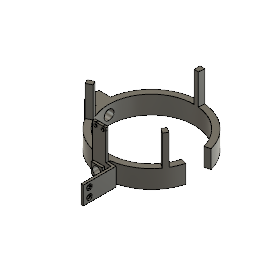
250-ml-band (Autodesk Fusion 360 design; units mm, degrees)
Autodesk Fusion 360 part; units mm, degrees
note: some values were not read from the file. Set by a fixed rule: which sketch regions a step uses.
sketch "Sketch1" plane through (0, 0, 0) normal (0, 1, 0) x (1, 0, 0)
  circle A0 centre (0, 0) radius 35
  circle A1 centre (0, 0) radius 40
  dimension "d1" = 70
  dimension "d2" = 5
  measures "d1" diameter of A0
extrude "Extrude1" add sketch "Sketch1" along normal blind 15
sketch "Sketch4" plane through (0, 15, 0) normal (0, 1, 0) x (-1, 0, 0)
  circle A0 centre (0, 0) radius 35
  circle A1 centre (0, 0) radius 40
  line L0 (0, 0) -> (0, -40)
  line L1 (0, 0) -> (-4.1811, -39.7809)
  line L2 (0, 0) -> (40, 0) construction
  dimension "d5" = 96
  dimension "d6" = 40
  measures "d5" angle of L1 L2
  measures "d6" distance of A0.centre L1.end
extrude "Extrude2" add sketch "Sketch4" along normal blind 25 contours A0 A1 L0 L1 picked at (-1.8026, -38.2856)
sketch "Sketch5" plane through (0, 15, 0) normal (0, 1, 0) x (-1, 0, 0)
  line L0 (0, -35) -> (0, -40)
  arc A0 (0, -40) -> (-4.1811, -39.7809) centre (0, 0) ccw
  line L1 (-4.1811, -39.7809) -> (-3.6585, -34.8083)
  arc A1 (0, -35) -> (-3.6585, -34.8083) centre (0, 0) ccw
  line L2 (0, 0) -> (-38.637, 10.3528)
  line L3 (0, 0) -> (40, 0) construction
  line L4 (0, 0) -> (-38.637, -10.3528)
  line L5 (0, 0) -> (-40, 0) construction
  dimension "d9" = 165
  dimension "d10" = 40
  dimension "d11" = 15
  dimension "d12" = 40
  measures "d9" angle of L2 L3
  measures "d10" distance of A0.centre L2.end
  measures "d11" angle of L4 L5
  measures "d12" distance of A0.centre L4.end
extrude "Extrude3" cut sketch "Sketch5" against normal blind 15 contours A0 A1 L2 L4
sketch "Sketch6" plane through (0, 15, 0) normal (0, 1, 0) x (-1, 0, 0)
  line L0 (-38.637, 10.3528) -> (-33.8074, 9.0587)
  arc A0 (0, -35) -> (-33.8074, 9.0587) centre (0, 0) ccw
  line L1 (0, -35) -> (0, -40)
  arc A1 (0, -40) -> (-38.637, 10.3528) centre (0, 0) ccw
  line L2 (0, 0) -> (-34.641, 20)
  line L3 (0, 0) -> (-40, 0) construction
  line L4 (0, 0) -> (-32.3607, 23.5114)
  line L5 (0, 0) -> (40, 0) construction
  dimension "d15" = 30
  dimension "d16" = 40
  dimension "d17" = 144
  dimension "d18" = 40
  measures "d15" angle of L2 L3
  measures "d16" distance of A0.centre L2.end
  measures "d17" angle of L4 L5
  measures "d18" distance of A0.centre L4.end
extrude "Extrude4" add sketch "Sketch6" along normal blind 25 contours A0 A1 L2 L4
sketch "Sketch7" plane through (0, 15, 0) normal (0, 1, 0) x (-1, 0, 0)
  line L0 (-32.3607, 23.5114) -> (-28.3156, 20.5725)
  arc A0 (0, -35) -> (-28.3156, 20.5725) centre (0, 0) ccw
  line L1 (0, -35) -> (0, -40)
  arc A1 (0, -40) -> (-32.3607, 23.5114) centre (0, 0) ccw
  line L2 (0, 0) -> (34.641, 20)
  line L3 (0, 0) -> (40, 0) construction
  line L4 (0, 0) -> (36.5418, 16.2695)
  line L5 (0, 0) -> (40, 0) construction
  dimension "d21" = 30
  dimension "d22" = 24
  dimension "d23" = 40
  measures "d21" angle of L2 L3
  measures "d22" angle of L4 L5
  measures "d23" distance of A0.centre L4.end
extrude "Extrude5" add sketch "Sketch7" along normal blind 25 contours A0 A1 L2 L4
sketch "Sketch8" plane through (0, 0, 0) normal (0, 1, 0) x (1, 0, 0)
  line L0 (0, 0) -> (-49.2, 0)
  line L1 (-49.2, 0) -> (-49.2, 6)
  line L2 (-49.2, 6) -> (-37.2, 6)
  line L3 (-37.2, 6) -> (-37.2, -6)
  line L4 (-37.2, -6) -> (-49.2, -6)
  line L5 (-49.2, -6) -> (-49.2, 6)
  dimension "d26" = 49.2
  dimension "d27" = 6
  dimension "d28" = 12
  dimension "d29" = 12
  measures "d26" distance of L0.start L0.end
  measures "d27" distance of L0.end L1.end
  measures "d28" distance of L1.end L2.end
  measures "d29" distance of L1.end L4.end
extrude "Extrude6" add sketch "Sketch8" along normal blind 15
sketch "Sketch9" plane through (0, 0, 0) normal (1, 0, 0) x (0, 0, -1)
  line L0 (0, 0) -> (0, 7.5)
  circle A0 centre (0, 7.5) radius 4
  dimension "d32" = 7.5
  dimension "d33" = 8
  measures "d32" distance of L0.start L0.end
  measures "d33" diameter of A0
extrude "Extrude7" cut sketch "Sketch9" against normal blind 47
sketch "Sketch10" plane through (0, 0, 0) normal (1, 0, 0) x (0, 0, -1)
  circle A0 centre (0, 7.5) radius 3.4
  point P0 (0, 7.5)
  dimension "d36" = 6.8
  measures "d36" diameter of A0
extrude "Extrude8" cut sketch "Sketch10" against normal blind 49.2
sketch "Sketch11" plane through (0, 0, 0) normal (0, 1, 0) x (1, 0, 0)
  line L0 (0, 0) -> (0, -43)
  line L1 (0, -43) -> (5.5, -43)
  line L2 (5.5, -43) -> (-5.5, -43)
  line L3 (-5.5, -43) -> (-5.5, -38)
  line L4 (-5.5, -38) -> (5.5, -38)
  line L5 (5.5, -38) -> (5.5, -43)
  dimension "d39" = 43
  dimension "d40" = 5.5
  dimension "d41" = 11
  dimension "d42" = 5
  measures "d39" distance of L0.start L0.end
  measures "d40" distance of L0.end L1.end
  measures "d41" distance of L1.end L2.end
  measures "d42" distance of L1.end L4.end
extrude "Extrude9" add sketch "Sketch11" along normal blind 15
sketch "Sketch12" plane through (0, 0, 43) normal (0, 0, 1) x (1, 0, 0)
  line L0 (-5.5, 0) -> (5.5, 0)
  line L1 (5.5, 0) -> (5.5, 15)
  line L2 (5.5, 15) -> (-5.5, 15)
  line L3 (-5.5, 15) -> (-5.5, 0)
  line L4 (0, 0) -> (0, 7.5)
  line L5 (4.5, 3) -> (-4.5, 3)
  line L6 (-4.5, 3) -> (-4.5, 12)
  line L7 (-4.5, 12) -> (4.5, 12)
  line L8 (4.5, 12) -> (4.5, 3)
  line L9 (4.5, 3) -> (-4.5, 12) construction
  line L10 (-4.5, 3) -> (4.5, 12) construction
  point P0 (0, 7.5)
  dimension "d45" = 7.5
  dimension "d46" = 9
  dimension "d47" = 9
  measures "d45" distance of L4.start P0
  measures "d46" distance of L6.end L7.end
  measures "d47" distance of L5.end L6.end
extrude "Extrude10" add sketch "Sketch12" along normal blind 2 contours L5 L6 L7 L8
sketch "Sketch13" plane through (0, 0, 45) normal (0, 0, 1) x (1, 0, 0)
  line L0 (4.5, 12) -> (-4.5, 12)
  line L1 (-4.5, 12) -> (-4.5, 3)
  line L2 (-4.5, 3) -> (4.5, 3)
  line L3 (4.5, 3) -> (4.5, 12)
  line L4 (0, 3) -> (0, 7.5)
  circle A0 centre (0, 7.5) radius 2
  circle A1 centre (0, 7.5) radius 3.5
  dimension "d50" = 4.5
  dimension "d51" = 4
  dimension "d54" = 7
  measures "d50" distance of L4.start L4.end
  measures "d51" diameter of A0
  measures "d54" diameter of A1
extrude "Extrude11" cut sketch "Sketch13" against normal blind 20 contours A0
extrude "Extrude12" cut sketch "Sketch13" against normal blind 9 contours A1
sketch "Sketch14" plane through (0, 15, 0) normal (0, 1, 0) x (-1, 0, 0)
  arc A0 (-5.5, 39.6201) -> (-32.3607, 23.5114) centre (0, 0) ccw
  line L0 (-32.3607, 23.5114) -> (-28.3156, 20.5725)
  arc A1 (30.3109, 17.5) -> (-28.3156, 20.5725) centre (0, 0) ccw
  line L1 (30.3109, 17.5) -> (34.641, 20)
  arc A2 (34.641, 20) -> (5.5, 39.6201) centre (0, 0) ccw
  line L2 (5.5, 39.6201) -> (5.5, 43)
  line L3 (5.5, 43) -> (-5.5, 43)
  line L4 (-5.5, 43) -> (-5.5, 39.6201)
  line L5 (5.5, 43) -> (-5.5, 43)
  line L6 (-5.5, 43) -> (-5.5, 41)
  line L7 (-5.5, 41) -> (5.5, 41)
  line L8 (5.5, 41) -> (5.5, 43)
  dimension "d57" = 11
  dimension "d58" = 2
  measures "d57" distance of L2.end L3.end
  measures "d58" distance of L2.end L7.end
extrude "Extrude13" add sketch "Sketch14" along normal blind 25 contours L2 L3 L4 L5 L6 L7 L8
sketch "Sketch15" plane through (5.5, 0, 0) normal (1, 0, 0) x (0, 0, -1)
  line L0 (-39.6201, 0) -> (-39.6201, 15)
  line L1 (-39.6201, 15) -> (-41, 15)
  line L2 (-41, 15) -> (-41, 40)
  line L3 (-41, 40) -> (-43, 40)
  line L4 (-43, 40) -> (-43, 0)
  line L5 (-43, 0) -> (-39.6201, 0)
  line L6 (-43, 0) -> (-41, 0)
  line L7 (-41, 0) -> (-41, 15)
  line L8 (-41, 15) -> (-43, 15)
  line L9 (-43, 15) -> (-43, 0)
extrude "Extrude14" add sketch "Sketch15" along normal blind 6.5 contours L4 L5 L6 L7 L8 L9
sketch "Sketch16" plane through (0, 0, 43) normal (0, 0, 1) x (1, 0, 0)
  line L0 (4.5, 12) -> (4.5, 3)
  line L1 (4.5, 3) -> (-4.5, 3)
  line L2 (-4.5, 3) -> (-4.5, 12)
  line L3 (-4.5, 12) -> (4.5, 12)
  line L4 (-5.5, 0) -> (12, 0)
  line L5 (12, 0) -> (12, 15)
  line L6 (12, 15) -> (5.5, 15)
  line L7 (5.5, 15) -> (5.5, 40)
  line L8 (5.5, 40) -> (-5.5, 40)
  line L9 (-5.5, 40) -> (-5.5, 0)
  line L10 (12, 15) -> (10, 15)
  line L11 (10, 15) -> (10, 0)
  line L12 (10, 0) -> (12, 0)
  line L13 (12, 0) -> (12, 15)
extrude "Extrude15" add sketch "Sketch16" along normal blind 25 contours L4 L5 L6 L10 L11 L12 L13
sketch "Sketch17" plane through (12, 0, 0) normal (1, 0, 0) x (0, 0, -1)
  line L0 (-68, 0) -> (-41, 0)
  line L1 (-41, 0) -> (-41, 15)
  line L2 (-41, 15) -> (-68, 15)
  line L3 (-68, 15) -> (-68, 0)
  line L4 (-68, 0) -> (-63, 0)
  line L5 (-63, 0) -> (-63, 4)
  circle A0 centre (-63, 4) radius 1.3
  dimension "d65" = 5
  dimension "d66" = 4
  dimension "d67" = 2.6
  measures "d65" distance of L0.start L4.end
  measures "d66" distance of L4.end L5.end
  measures "d67" diameter of A0
extrude "Extrude16" cut sketch "Sketch17" against normal blind 2 contours A0
sketch "Sketch18" plane through (12, 0, 0) normal (1, 0, 0) x (0, 0, -1)
  circle A0 centre (-63, 4) radius 1.3
  line L0 (-68, 0) -> (-41, 0)
  line L1 (-41, 0) -> (-41, 15)
  line L2 (-41, 15) -> (-68, 15)
  line L3 (-68, 15) -> (-68, 0)
  line L4 (-68, 15) -> (-63, 15)
  line L5 (-63, 15) -> (-63, 11)
  circle A1 centre (-63, 11) radius 1.3
  dimension "d70" = 5
  dimension "d71" = 4
  dimension "d72" = 2.6
  measures "d70" distance of L2.end L4.end
  measures "d71" distance of L4.end L5.end
  measures "d72" diameter of A1
extrude "Extrude17" cut sketch "Sketch18" against normal blind 2 contours A1
sketch "Sketch19" plane through (0, 0, 43) normal (0, 0, 1) x (1, 0, 0)
  line L0 (10, 0) -> (10, 15)
  line L1 (10, 15) -> (5.5, 15)
  line L2 (5.5, 15) -> (5.5, 40)
  line L3 (5.5, 40) -> (-5.5, 40)
  line L4 (-5.5, 40) -> (-5.5, 0)
  line L5 (-5.5, 0) -> (10, 0)
  line L6 (4.5, 12) -> (4.5, 3)
  line L7 (4.5, 3) -> (-4.5, 3)
  line L8 (-4.5, 3) -> (-4.5, 12)
  line L9 (-4.5, 12) -> (4.5, 12)
  line L10 (-5.5, 40) -> (-3, 40)
  line L11 (-3, 40) -> (-3, 37.5)
  circle A0 centre (-3, 37.5) radius 1.3
  dimension "d75" = 2.5
  dimension "d76" = 2.5
  dimension "d77" = 2.6
  measures "d75" distance of L3.end L10.end
  measures "d76" distance of L10.end L11.end
  measures "d77" diameter of A0
extrude "Extrude18" cut sketch "Sketch19" against normal blind 2 contours A0
sketch "Sketch20" plane through (0, 0, 43) normal (0, 0, 1) x (1, 0, 0)
  circle A0 centre (-3, 37.5) radius 1.3
  line L0 (10, 0) -> (10, 15)
  line L1 (10, 15) -> (5.5, 15)
  line L2 (5.5, 15) -> (5.5, 40)
  line L3 (5.5, 40) -> (-5.5, 40)
  line L4 (-5.5, 40) -> (-5.5, 0)
  line L5 (-5.5, 0) -> (10, 0)
  line L6 (4.5, 12) -> (4.5, 3)
  line L7 (4.5, 3) -> (-4.5, 3)
  line L8 (-4.5, 3) -> (-4.5, 12)
  line L9 (-4.5, 12) -> (4.5, 12)
  line L10 (5.5, 40) -> (3, 40)
  line L11 (3, 40) -> (3, 37.5)
  circle A1 centre (3, 37.5) radius 1.3
  dimension "d80" = 2.5
  dimension "d81" = 2.5
  dimension "d82" = 2.6
  measures "d80" distance of L2.end L10.end
  measures "d81" distance of L10.end L11.end
  measures "d82" diameter of A1
extrude "Extrude19" cut sketch "Sketch20" against normal blind 2 contours A1
sketch "Sketch21" plane through (12, 0, 0) normal (1, 0, 0) x (0, 0, -1)
  circle A0 centre (-63, 11) radius 1.3
  circle A1 centre (-63, 4) radius 1.3
  line L0 (-68, 0) -> (-41, 0)
  line L1 (-41, 0) -> (-41, 15)
  line L2 (-41, 15) -> (-68, 15)
  line L3 (-68, 15) -> (-68, 0)
  circle A2 centre (-63, 11) radius 2.2
  dimension "d85" = 4.4
  measures "d85" diameter of A2
extrude "Extrude20" cut sketch "Sketch21" against normal blind 1 contours A2
sketch "Sketch22" plane through (12, 0, 0) normal (1, 0, 0) x (0, 0, -1)
  circle A0 centre (-63, 11) radius 2.2
  circle A1 centre (-63, 4) radius 1.3
  line L0 (-68, 0) -> (-41, 0)
  line L1 (-41, 0) -> (-41, 15)
  line L2 (-41, 15) -> (-68, 15)
  line L3 (-68, 15) -> (-68, 0)
  circle A2 centre (-63, 4) radius 2.2
  dimension "d88" = 4.4
  measures "d88" diameter of A2
extrude "Extrude21" cut sketch "Sketch22" against normal blind 1 contours A2
sketch "Sketch23" plane through (0, 0, 41) normal (0, 0, -1) x (-1, 0, 0)
  circle A0 centre (-3, 37.5) radius 1.3
  circle A1 centre (3, 37.5) radius 1.3
  line L0 (-5.5, 15) -> (5.5, 15)
  line L1 (5.5, 15) -> (5.5, 40)
  line L2 (5.5, 40) -> (-5.5, 40)
  line L3 (-5.5, 40) -> (-5.5, 15)
  circle A2 centre (3, 37.5) radius 2.2
  dimension "d91" = 4.4
  measures "d91" diameter of A2
extrude "Extrude22" cut sketch "Sketch23" against normal blind 1 contours A2
sketch "Sketch24" plane through (0, 0, 41) normal (0, 0, -1) x (-1, 0, 0)
  circle A0 centre (3, 37.5) radius 2.2
  circle A1 centre (-3, 37.5) radius 1.3
  line L0 (-5.5, 15) -> (5.5, 15)
  line L1 (5.5, 15) -> (5.5, 40)
  line L2 (5.5, 40) -> (-5.5, 40)
  line L3 (-5.5, 40) -> (-5.5, 15)
  circle A2 centre (-3, 37.5) radius 2.2
  dimension "d94" = 4.4
  measures "d94" diameter of A2
extrude "Extrude23" cut sketch "Sketch24" against normal blind 1 contours A2
